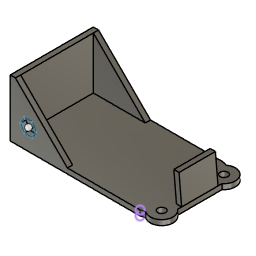
9v holder (Autodesk Fusion 360 design; units mm, degrees)
Autodesk Fusion 360 part; units mm, degrees
note: some values were not read from the file. Set by a fixed rule: which sketch regions a step uses.
sketch "Sketch1" plane through (0, 0, 0) normal (0, 0, 1) x (1, 0, 0)
  line L0 (25, 16) -> (-25, 16)
  line L1 (-25, 16) -> (-25, -16)
  line L2 (-25, -16) -> (25, -16)
  line L3 (25, -16) -> (25, 16)
  line L4 (25, 16) -> (-25, -16) construction
  line L5 (-25, 16) -> (25, -16) construction
  dimension "d1" = 50
  dimension "d2" = 32
  constraint horizontal L0
  constraint perpendicular L0 L1
  constraint parallel L0 L2
  constraint parallel L1 L3
  constraint coincident L4 origin
  constraint coincident L5 origin
  measures "d1" distance of L1.end L2.end
  measures "d2" distance of L0.end L1.end
extrude "Extrude1" add sketch "Sketch1" along normal blind 2
sketch "Sketch2" plane through (0, 0, 2) normal (0, 0, 1) x (-1, 0, 0)
  line L0 (-25, 16) -> (-25, -16)
  line L1 (-25, -16) -> (25, -16)
  line L2 (25, -16) -> (25, 16)
  line L3 (25, 16) -> (-25, 16)
  line L4 (23, 14) -> (-23, 14)
  line L5 (-23, 14) -> (-23, -14)
  line L6 (-23, -14) -> (23, -14)
  line L7 (23, -14) -> (23, 14)
  line L8 (-25, 16) -> (25, 16)
  line L9 (25, 16) -> (25, -16)
  line L10 (25, -16) -> (-25, -16)
  line L11 (-25, -16) -> (-25, 16)
  line L12 (-25, 16) -> (25, -16) construction
  line L13 (25, 16) -> (-25, -16) construction
  dimension "d5" = -2
  constraint horizontal L8
  constraint perpendicular L8 L9
  constraint parallel L8 L10
  constraint parallel L9 L11
  constraint coincident L12 origin
  constraint coincident L13 origin
  constraint coincident L0.start L3.end
extrude "Extrude2" add sketch "Sketch2" along normal blind 20
sketch "Sketch3" plane through (0, -16, 0) normal (0, -1, 0) x (1, 0, 0)
  line L0 (-25, 0) -> (25, 0)
  line L1 (25, 0) -> (25, 22)
  line L2 (25, 22) -> (-25, 22)
  line L3 (-25, 22) -> (-25, 0)
  line L4 (-25, 22) -> (-23, 22)
  line L5 (-25, 0) -> (-25, 2)
  line L6 (-25, 2) -> (25, 2)
  line L7 (-23, 22) -> (-3, 2)
  line L8 (-23, 22) -> (25, 22)
  line L9 (25, 2) -> (25, 22)
  constraint coincident L2.end L3.start
  constraint coincident L2 L4.end
  constraint perpendicular L3 L4
  constraint coincident L0.start L3.end
  constraint coincident L3 L5.end
  constraint perpendicular L5 L6
  constraint coincident L6 L7.end
  constraint coincident L1.end L2.start
  constraint coincident L1 L6.end
extrude "Extrude3" cut sketch "Sketch3" against normal blind 40 contours L1 L2 L6 L7 L8 L9
sketch "Sketch4" plane through (0, 0, 2) normal (0, 0, 1) x (-1, 0, 0)
  line L0 (3, -14) -> (23, -14)
  line L1 (23, -14) -> (23, 14)
  line L2 (23, 14) -> (3, 14)
  line L3 (3, 14) -> (3, 16)
  line L4 (3, 16) -> (-25, 16)
  line L5 (23, 0) -> (-24, 0)
  line L6 (-24, 0) -> (-32, 0)
  line L7 (-32, 0) -> (-32, -14)
  line L8 (-32, -14) -> (-25, -16)
  line L9 (-32, 0) -> (-32, 14)
  line L10 (-32, 14) -> (-25, 16)
  line L11 (-25, -16) -> (3, -16)
  line L12 (3, -16) -> (3, -14)
  line L13 (-25, 16) -> (-25, -16)
  constraint midpoint L1 L5.start
  constraint perpendicular L6 L7
  constraint coincident L8.end L11.start
  constraint perpendicular L6 L9
  constraint coincident L4.end L10.end
extrude "Extrude4" add sketch "Sketch4" against normal blind 2 contours L6 L7 L8 L13 | L6 L9 L10 L13
sketch "Sketch5" plane through (0, 0, 2) normal (0, 0, 1) x (-1, 0, 0)
  line L0 (3, -14) -> (23, -14)
  line L1 (23, -14) -> (23, 14)
  line L2 (23, 14) -> (3, 14)
  line L3 (3, 14) -> (3, 16)
  line L4 (3, 16) -> (-25, 16)
  line L5 (-32, 10) -> (-28, 10)
  line L6 (-28, 10) -> (-28, -10)
  line L7 (-28, -10) -> (-32, -10)
  line L8 (-32, -10) -> (-32, 10)
  line L9 (-32, -10) -> (-32, -7)
  line L10 (-32, 10) -> (-32, 7)
  line L11 (-32, 7) -> (-28, 7)
  line L12 (-32, -7) -> (-28, -7)
  line L13 (-25, -16) -> (3, -16)
  line L14 (3, -16) -> (3, -14)
  line L15 (-25, 16) -> (-32, 14)
  line L16 (-32, 14) -> (-32, -14)
  line L17 (-32, -14) -> (-25, -16)
  dimension "d45" = 20
  constraint horizontal L5
  constraint vertical L6
  constraint horizontal L7
  constraint vertical L8
  constraint coincident L8 L9.end
  constraint coincident L8 L10.end
  constraint coincident L6 L11.end
  constraint perpendicular L6 L11
  constraint coincident L6 L12.end
  constraint perpendicular L6 L12
  measures "d45" distance of L5.start L7.end
extrude "Extrude5" add sketch "Sketch5" along normal blind 11 contours L6 L8 L11 L12 L16
sketch "Sketch6" plane through (0, -7, 0) normal (0, -1, 0) x (1, 0, 0)
  line L0 (28, 2) -> (32, 2)
  line L1 (32, 2) -> (32, 13)
  line L2 (32, 13) -> (28, 13)
  line L3 (28, 13) -> (28, 2)
  line L4 (32, 2) -> (30, 2)
  line L5 (29, 13) -> (30, 2)
  line L6 (32, 2) -> (31, 13)
  line L7 (29, 13) -> (31, 13)
  line L8 (28, 2) -> (32, 2)
  line L9 (32, 2) -> (32, 13)
  line L10 (32, 13) -> (28, 13)
  line L11 (28, 13) -> (28, 2)
  dimension "d14" = 2
  constraint coincident L0.end L1.start
  constraint midpoint L0 L4.end
  constraint coincident L2 L5.start
  constraint coincident L2 L6.end
  constraint parallel L5 L6
  measures "d14" distance of L0.end L4.end
extrude "Extrude6" cut sketch "Sketch6" against normal blind 20 contours L0 L2 L3 L5 L8 L10 L11 | L1 L2 L6 L9 L10
sketch "Sketch7" plane through (0, -16, 0) normal (0, -1, 0) x (1, 0, 0)
  line L0 (25, 2) -> (-3, 2)
  line L1 (-3, 2) -> (-23, 22)
  line L2 (-23, 22) -> (-25, 22)
  line L3 (-25, 22) -> (-25, 0)
  line L4 (-25, 0) -> (25, 0)
  line L5 (-15, 8) -> (-16.5, 10.5981)
  line L6 (-16.5, 10.5981) -> (-19.5, 10.5981)
  line L7 (-19.5, 10.5981) -> (-21, 8)
  line L8 (-21, 8) -> (-19.5, 5.4019)
  line L9 (-19.5, 5.4019) -> (-16.5, 5.4019)
  line L10 (-16.5, 5.4019) -> (-15, 8)
  point P0 (-18, 8)
extrude "Extrude8" cut sketch "Sketch7" against normal blind 29
sketch "Sketch9" plane through (0, 0, 0) normal (0, 0, -1) x (1, 0, 0)
  line L0 (25, 16) -> (-25, 16)
  line L1 (-25, 16) -> (-25, -16)
  line L2 (-25, -16) -> (25, -16)
  line L3 (25, -16) -> (32, -14)
  line L4 (32, -14) -> (32, 14)
  line L5 (32, 14) -> (25, 16)
  line L6 (-25, 0) -> (32, 0) construction
  line L7 (31.5, 14.5) -> (-24.5, 14.5) construction
  line L8 (-24.5, 14.5) -> (-24.5, -14.5) construction
  line L9 (-24.5, -14.5) -> (31.5, -14.5) construction
  line L10 (31.5, -14.5) -> (31.5, 14.5) construction
  line L11 (31.5, 14.5) -> (-24.5, -14.5) construction
  line L12 (-24.5, 14.5) -> (31.5, -14.5) construction
  line L13 (30.8, -14.5) -> (30.8, 14.5) construction
  line L14 (31.5, 13.5) -> (-24.5, 13.5) construction
  circle A0 centre (29.3, 12) radius 1.5
  circle A1 centre (29.3, -12) radius 1.5
  line L15 (3.5, 0) -> (3.5, 14.5) construction
  line L16 (3.5, 0) -> (3.5, -14.5) construction
  point P0 (3.5, 0)
  dimension "d38" = 56
  dimension "d39" = 29
  dimension "d40" = -0.7
  dimension "d41" = -1
  dimension "d42" = 1.5
  constraint midpoint L1 L6.start
  constraint midpoint L4 L6.end
  constraint horizontal L7
  constraint perpendicular L7 L8
  constraint parallel L7 L9
  constraint parallel L8 L10
  constraint coincident L11 P0
  constraint coincident L12 P0
  constraint midpoint L6 P0
  constraint tangent L14 A0
  constraint tangent L13 A0
  constraint symmetric L6 A0 A1
  constraint coincident P0 L15.start
  constraint midpoint L7 L15.end
  constraint midpoint L9 L16.end
  measures "d4" distance of L8.end L9.end
  measures "d4" distance of L7.end L8.end
  measures "d42" radius of A0
extrude "Extrude10" cut sketch "Sketch9" against normal blind 30 contours A0 | A1
sketch "Sketch10" plane through (0, 0, 2) normal (0, 0, 1) x (-1, 0, 0)
  circle A0 centre (-29.3, -12) radius 1.5
  circle A1 centre (-29.3, 12) radius 1.5
  line L0 (-30, -7) -> (-32, -7)
  line L1 (-32, -7) -> (-32, -14)
  line L2 (-32, -14) -> (-25, -16)
  line L3 (-25, 16) -> (-32, 14)
  line L4 (-32, 7) -> (-30, 7)
  line L5 (-30, 7) -> (-30, -7)
  arc A2 (-26.682, 15.5194) -> (-31.5, 8.2053) centre (-29.3, 12) ccw
  arc A3 (-32, -8.5431) -> (-26.682, -15.5194) centre (-29.3, -12) ccw
  line L6 (-25, -16) -> (3, -16)
  line L7 (3, -16) -> (3, -14)
  line L8 (3, -14) -> (23, -14)
  line L9 (23, -14) -> (23, 14)
  line L10 (23, 14) -> (3, 14)
  line L11 (3, 14) -> (3, 16)
  line L12 (3, 16) -> (-25, 16)
  line L13 (-32, 14) -> (-32, 7)
  dimension "d46" = 4.3863
  dimension "d47" = 4.3863
  constraint concentric A1 A2
  constraint coincident L3 A2.start
  constraint concentric A0 A3
  constraint coincident L2 A3.end
  constraint coincident L1 A3.start
  measures "d46" radius of A2
  measures "d47" radius of A3
extrude "Extrude11" add sketch "Sketch10" against normal blind 2 contours L1 L2 A3 | L3 A2 L13
